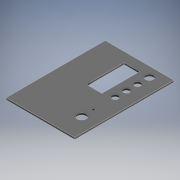
# Autodesk Inventor part: component box cover
Saved by Autodesk Inventor 2021 (Build 250183000, 183)
## iProperties
Created: 2023-01-12
Part Number: component box cover
Material: Generic
Document SubType Name: Modeling
Designer: boyle
Density: 1 g/cm^3
Appearance: Default
Author: boyle
Autodesk Inventor part; units mm, degrees
ref_plane "YZ Plane" through (0, 0, 0) normal (1, 0, 0) x (0, 1, 0)
ref_plane "XZ Plane" through (0, 0, 0) normal (0, 1, 0) x (-1, 0, 0)
ref_plane "XY Plane" through (0, 0, 0) normal (0, 0, 1) x (1, 0, 0)
sketch "Sketch1" plane through (0, 0, 0) normal (0, 1, 0) x (-1, 0, 0)
  line L0 (0, 0) -> (-177.8, 0)
  line L1 (-177.8, 0) -> (-177.8, 256.54)
  line L2 (-177.8, 256.54) -> (0, 256.54)
  line L3 (0, 256.54) -> (0, 0)
  dimension "d0" = 177.8
  dimension "d1" = 256.54
  constraints: 8 end point, 2 parallel, 1 horizontal, 1 perpendicular
  measures "d0" distance of L1.end L2.end
  measures "d1" distance of L0.end L1.end
extrude "Extrusion1" add sketch "Sketch1" along normal blind 4.826
sketch "Sketch2" plane through (0, 4.826, 0) normal (0, 1, 0) x (1, 0, 0)
  line L0 (0, -256.54) -> (177.8, -256.54) projected
  line L1 (177.8, -256.54) -> (177.8, 0) projected
  line L2 (177.8, 0) -> (0, 0) projected
  line L3 (0, 0) -> (0, -256.54) projected
  line L4 (0, -256.54) -> (177.8, -256.54) projected
  line L5 (177.8, -256.54) -> (177.8, 0) projected
  line L6 (88.9, -256.54) -> (177.8, -256.54)
  line L7 (177.8, -256.54) -> (177.8, -128.27)
  line L8 (177.8, -128.27) -> (88.9, -128.27)
  line L9 (88.9, -128.27) -> (88.9, -256.54)
  line L10 (0, -256.54) -> (177.8, -256.54) projected
  line L11 (88.9, -256.54) -> (0, -256.54)
  line L12 (0, 0) -> (0, -256.54) projected
  line L13 (177.8, 0) -> (0, 0) projected
  line L14 (0, 0) -> (0, -256.54) projected
  line L15 (0, -128.27) -> (50.8, -128.27)
  line L16 (50.8, -128.27) -> (50.8, 0)
  line L17 (50.8, -64.135) -> (177.8, -64.135)
  line L18 (146.05, -51.2875) -> (139.7, -51.2875)
  line L19 (139.7, -64.135) -> (139.7, -228.6)
  line L20 (139.7, -51.2875) -> (139.7, 0)
  line L21 (139.7, 0) -> (139.7, -12.7)
  line L22 (139.7, 0) -> (139.7, -25.4)
  circle A0 centre (139.7, -25.4) radius 10
  line L23 (139.7, -25.4) -> (139.7, -50.8)
  line L24 (139.7, -35.4) -> (139.7, -60.8)
  circle A1 centre (139.7, -56.0525) radius 8.1
  line L25 (139.7, -47.9525) -> (139.7, -56.0525)
  line L26 (139.7, -64.1525) -> (139.7, -84.9525)
  circle A2 centre (139.7, -84.9525) radius 8.1
  line L27 (139.7, -93.0525) -> (139.7, -113.8551)
  circle A3 centre (139.7, -113.8551) radius 8.1
  line L28 (139.7, -228.6) -> (139.7, -200.66)
  circle A4 centre (139.7, -200.66) radius 11.5
  line L29 (114.3, -200.66) -> (139.7, -200.66)
  line L30 (114.0965, -24.8721) -> (73.8465, -24.8721)
  line L31 (73.8465, -24.8721) -> (73.8465, -122.8721)
  line L32 (73.8465, -122.8721) -> (114.0965, -122.8721)
  line L33 (114.0965, -122.8721) -> (114.0965, -24.8721)
  line L34 (139.7, -200.66) -> (139.7, -175.26)
  line L35 (139.7, -175.26) -> (139.7, -170.18)
  circle A5 centre (139.7, -170.18) radius 3.1
  dimension "d14" = 20
  dimension "d18" = 16.2
  dimension "d9" = 50.8
  dimension "d13" = 25.4
  dimension "d17" = 25.4
  dimension "d19" = 8.1
  dimension "d20" = 20.8
  dimension "d22" = 20.8026
  dimension "d23" = 27.94
  dimension "d24" = 23
  dimension "d27" = 25.4
  dimension "d28" = 40.25
  dimension "d29" = 98
  dimension "d30" = 25.4
  dimension "d31" = 5.08
  dimension "d32" = 6.2
  constraints: 52 end point, 9 point on line, 5 coincident, 5 perpendicular, 4 horizontal, 4 midpoint, 4 parallel, 3 centre point, 3 vertical alignment, 1 collinear, 1 vertical, 7 other
  measures "d9" distance of L15.start L15.end
  measures "d13" distance of L20.end L22.end
  measures "d17" distance of L24.end L24.start
  measures "d19" distance of L25.start L25.end
  measures "d20" distance of L26.start L26.end
  measures "d22" distance of L27.start L27.end
  measures "d23" distance of L19.end L28.end
  measures "d24" diameter of A4
  measures "d27" distance of L29.start L29.end
  measures "d28" distance of L32.end L31.end
  measures "d29" distance of L31.end L30.end
  measures "d30" distance of L29.end L34.end
  measures "d31" distance of L34.end L35.end
  measures "d32" diameter of A5
extrude "Extrusion3" cut sketch "Sketch2" against normal blind 25.4 contours A3 L19 | L19 A3 | L31 L30 L33 L17 | L17 L33 L32 L31 | A1 L19 L17 | L17 A1 | L19 A1 L17 | A2 L19 | L19 A2 | A0 L20 | L20 A0 | A5 L19 | L19 A5 | A4 L19 | L19 L29 A4 | L19 A4 L29
body "Solid1"
